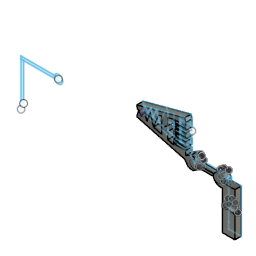
CompliantHands v5 (Autodesk Fusion 360 design; units mm, degrees)
Autodesk Fusion 360 part; units mm, degrees
sketch "Sketch1" plane through (0, 0, 0) normal (0, 1, 0) x (1, 0, 0)
  line L0 (0, 0) -> (19.3185, 5.1764)
  line L1 (0, 0) -> (0.7765, -2.8978)
  line L2 (20.095, 2.2786) -> (19.3185, 5.1764)
  line L3 (0.7765, -2.8978) -> (3.6742, -2.1213)
  line L4 (3.6742, -2.1213) -> (6.572, -1.3449)
  line L5 (6.572, -1.3449) -> (9.4698, -0.5684)
  line L6 (9.4698, -0.5684) -> (12.3676, 0.2081)
  line L7 (12.3676, 0.2081) -> (15.2653, 0.9845)
  line L8 (15.2653, 0.9845) -> (18.1631, 1.761)
  line L9 (20.095, 2.2786) -> (18.1631, 1.761)
  line L10 (12.3676, -8.3553) -> (15.2653, -9.1317)
  line L11 (9.4723, -7.5695) -> (12.3676, -8.3553)
  line L12 (15.2653, -9.1317) -> (18.1631, -9.9082)
  line L13 (0, -8.1472) -> (19.3185, -13.3236)
  line L14 (0.7833, -5.2241) -> (3.6811, -6.0006)
  line L15 (6.5789, -6.777) -> (9.4723, -7.5695)
  line L16 (3.6811, -6.0006) -> (6.5789, -6.777)
  line L17 (20.095, -10.4258) -> (18.1631, -9.9082)
  line L18 (20.095, -10.4258) -> (19.3185, -13.3236)
  line L19 (20.095, 2.2786) -> (20.095, -10.4258)
  line L20 (19.3185, 5.1764) -> (38.637, 10.3528)
  line L21 (20.095, 2.2786) -> (39.4135, 7.455)
  line L22 (39.4135, 7.455) -> (38.637, 10.3528)
  line L23 (20.095, -10.4258) -> (39.4135, -15.6022)
  line L24 (19.3185, -13.3236) -> (38.637, -18.5)
  line L25 (38.637, -18.5) -> (39.4135, -15.6022)
  line L26 (20.095, 2.2786) -> (24.9246, 3.5727)
  line L27 (24.9246, 3.5727) -> (24.9246, -4.0736)
  line L28 (24.9246, -4.0736) -> (24.9246, -11.7199)
  line L29 (20.095, -4.0736) -> (22.095, -4.0736)
  line L30 (24.9246, -4.0736) -> (24.9246, -6.0736)
  line L31 (22.095, -4.0736) -> (24.9246, -6.0736)
  line L32 (24.9246, -4.0736) -> (24.9246, -2.0736)
  line L33 (22.095, -4.0736) -> (24.9246, -2.0736)
  line L34 (39.4135, 7.455) -> (39.4135, 4.8668)
  line L35 (39.4135, 4.8668) -> (29.7542, 4.8668)
  line L36 (39.4135, -15.6022) -> (39.4135, -13.014)
  line L37 (39.4135, -13.014) -> (29.7542, -13.014)
  line L38 (39.4135, 7.455) -> (43.713, 4.9027)
  line L39 (38.637, 10.3528) -> (41.5877, 14.3893)
  line L40 (41.5877, 14.3893) -> (43.713, 4.9027)
  line L41 (39.4135, 0.8668) -> (38.4135, 0.8668)
  line L42 (39.4135, 0.8668) -> (39.4135, 1.8668)
  line L43 (39.4135, 1.8668) -> (29.7542, 1.8668)
  line L44 (29.7542, 1.8668) -> (29.7542, 0.8668)
  line L45 (29.7542, 0.8668) -> (38.4135, 0.8668)
  line L46 (29.7542, 1.8668) -> (29.7542, 4.8668)
  line L47 (29.7542, 4.8668) -> (30.7542, 4.8668)
  line L48 (30.7542, 4.8668) -> (30.7542, 1.8668)
  line L49 (30.7542, 4.8668) -> (39.4135, 4.8668)
  line L50 (39.4135, 4.8668) -> (39.4135, 5.0729)
  circle A0 centre (45.9703, 10.3897) radius 3.4023
  line L51 (46.28, 5.4777) -> (43.713, 4.9027)
  line L52 (41.5877, 14.3893) -> (44.1548, 14.9643)
  spline S0 degree 5 poles (47.6847, 13.3285) (47.6048, 13.4012) (47.4459, 13.5431) (47.2099, 13.746) (46.8999, 13.9959) (46.5209, 14.2717) (46.1512, 14.5071) (45.7919, 14.6983) (45.4434, 14.8421) (45.106, 14.9387) (44.7788, 14.9908) (44.5247, 14.9995) (44.3382, 14.9886) (44.2156, 14.9737) (44.1548, 14.9643) knots 0 0 0 0 0 0 0.1 0.2 0.3 0.4 0.5 0.6 0.7 0.8 0.9 1 1 1 1 1 1
  spline S1 degree 5 poles (48.7311, 8.4013) (48.6822, 8.304) (48.5842, 8.1125) (48.4374, 7.835) (48.2415, 7.4848) (47.9966, 7.0826) (47.7516, 6.7194) (47.5065, 6.3991) (47.2614, 6.1252) (47.0161, 5.8979) (46.7708, 5.7146) (46.5745, 5.6007) (46.4273, 5.5326) (46.3291, 5.4948) (46.28, 5.4777) knots 0 0 0 0 0 0 0.1 0.2 0.3 0.4 0.5 0.6 0.7 0.8 0.9 1 1 1 1 1 1
  circle A1 centre (45.9703, 10.3897) radius 3.3
  line L53 (45.9703, 10.3897) -> (45.9703, 9.3897)
  line L54 (45.9703, 9.3897) -> (70.9703, 9.3897)
  line L55 (70.9703, 9.3897) -> (70.9703, 10.3897)
  line L56 (45.9703, 10.3897) -> (45.9703, 11.3897)
  line L57 (45.9703, 11.3897) -> (70.9703, 11.3897)
  line L58 (70.9703, 11.3897) -> (70.9703, 10.3897)
  line L59 (39.4135, 4.8668) -> (39.4135, 3.8668)
  line L60 (39.4135, 3.8668) -> (30.7542, 3.8668)
  line L61 (39.4135, 1.8668) -> (39.4135, -1.1332)
  line L62 (39.4135, -1.1332) -> (39.4135, -2.1332)
  line L63 (39.4135, -2.1332) -> (29.7542, -2.1332)
  line L64 (29.7542, -2.1332) -> (29.7542, -1.1332)
  line L65 (29.7542, -1.1332) -> (39.4135, -1.1332)
  line L66 (39.4135, -2.1332) -> (38.4135, -2.1332)
  line L67 (38.4135, -2.1332) -> (38.4135, 0.8668)
  line L68 (29.7542, -2.1332) -> (29.7542, -5.1332)
  line L69 (29.7542, -5.1332) -> (39.4135, -5.1332)
  line L70 (39.4135, -5.1332) -> (39.4135, -4.1332)
  line L71 (39.4135, -4.1332) -> (29.7542, -4.1332)
  line L72 (29.7542, -2.1332) -> (30.7542, -2.1332)
  line L73 (30.7542, -2.1332) -> (30.7542, -5.1332)
  line L74 (39.4135, -5.1332) -> (39.4135, -8.1332)
  line L75 (39.4135, -8.1332) -> (29.7542, -8.1332)
  line L76 (29.7542, -8.1332) -> (29.7542, -7.1332)
  line L77 (29.7542, -7.1332) -> (39.4135, -7.1332)
  line L78 (39.4135, -5.1332) -> (38.4135, -5.1332)
  line L79 (38.4135, -5.1332) -> (38.4135, -7.1332)
  line L80 (29.7542, -8.1332) -> (29.7542, -11.1332)
  line L81 (29.7542, -11.1332) -> (39.4135, -11.1332)
  line L82 (39.4135, -11.1332) -> (39.4135, -10.1332)
  line L83 (39.4135, -10.1332) -> (29.7542, -10.1332)
  line L84 (29.7542, -8.1332) -> (30.7542, -8.1332)
  line L85 (30.7542, -8.1332) -> (30.7542, -10.1332)
  line L86 (39.4135, -11.1332) -> (39.4135, -13.014)
  line L87 (39.4135, -11.1332) -> (38.4135, -11.1332)
  line L88 (38.4135, -11.1332) -> (38.4135, -13.014)
  line L89 (68.9703, 41.3897) -> (68.9703, 11.3897)
  line L90 (-98.0297, 41.3897) -> (-98.0297, 46.3897)
  line L91 (-98.0297, 41.3897) -> (-98.0297, 11.3897)
  line L92 (-98.0297, 11.3897) -> (-96.0297, 11.3897)
  line L93 (-96.0297, 11.3897) -> (-96.0297, 41.3897)
  line L94 (-98.0297, 11.3897) -> (-98.0297, 9.3897)
  line L95 (-98.0297, 9.3897) -> (-68.0297, 9.3897)
  line L96 (-68.0297, 9.3897) -> (-68.0297, 11.3897)
  line L97 (-68.0297, 11.3897) -> (-96.0297, 11.3897)
  circle A2 centre (-68.0297, 10.3897) radius 3.3
  line L98 (0.7833, -5.2241) -> (0.9425, -5.2668)
  line L99 (0.7833, -5.2241) -> (0, -8.1472)
  line L100 (1.6898, -5.2715) -> (0.7765, -2.8978)
  line L101 (1.6898, -5.2715) -> (3.6742, -2.1213)
  line L102 (3.769, -2.3626) -> (6.2428, -6.687)
  line L103 (3.769, -2.3626) -> (1.7888, -5.4936)
  line L104 (6.3223, -6.3567) -> (3.8459, -2.0753)
  line L105 (8.0209, -0.9566) -> (6.3223, -6.3567)
  line L106 (8.1279, -1.3139) -> (10.9199, -7.9624)
  line L107 (8.1279, -1.3139) -> (6.4337, -6.7381)
  line L108 (10.9903, -7.6343) -> (13.4864, 0.5078)
  line L109 (10.9903, -7.6343) -> (8.2001, -0.9086)
  line L110 (13.5902, 0.1178) -> (11.0545, -7.9989)
  line L111 (13.5902, 0.1178) -> (17.6214, -9.763)
  line L112 (68.9703, 10.3897) -> (68.9703, 15.3897)
  line L113 (68.9703, 10.3897) -> (68.9703, 5.3897)
  line L114 (68.9703, 10.3897) -> (64.9703, 10.3897)
  circle A3 centre (64.9703, 10.3897) radius 3.4
  circle A4 centre (64.9703, 10.3897) radius 3.3
  spline S2 degree 5 poles (68.9703, 5.3897) (68.8004, 5.3839) (68.4641, 5.3773) (67.9703, 5.3823) (67.3336, 5.4196) (66.5762, 5.5207) (65.8611, 5.6813) (65.192, 5.9068) (64.5715, 6.2007) (63.9983, 6.5614) (63.4693, 6.9844) (63.0786, 7.3687) (62.8027, 7.6811) (62.6263, 7.8999) (62.54, 8.012) knots 0 0 0 0 0 0 0.1 0.2 0.3 0.4 0.5 0.6 0.7 0.8 0.9 1 1 1 1 1 1
  spline S3 degree 5 poles (68.9703, 15.3897) (68.7911, 15.4037) (68.4369, 15.4261) (67.9187, 15.4426) (67.2541, 15.4299) (66.4705, 15.3522) (65.7385, 15.2068) (65.0627, 14.9875) (64.4466, 14.6899) (63.8891, 14.3155) (63.3861, 13.8693) (63.0241, 13.4595) (62.7739, 13.1241) (62.6164, 12.8884) (62.54, 12.7674) knots 0 0 0 0 0 0 0.1 0.2 0.3 0.4 0.5 0.6 0.7 0.8 0.9 1 1 1 1 1 1
  line L115 (68.9703, 5.3897) -> (70.9703, 9.3897)
  line L116 (68.9703, 11.3897) -> (73.9703, 11.3897)
  line L117 (68.9703, 41.3897) -> (68.9703, 46.3897)
  line L118 (68.9703, 46.3897) -> (78.9703, 46.3897)
  line L119 (78.9703, 46.3897) -> (78.9703, 11.3897)
  line L120 (78.9703, 11.3897) -> (73.9703, 11.3897)
  line L121 (73.9703, 28.6756, 0) -> (73.9703, 28.6756, -2.5)
  spline S4 degree 5 poles (78.9703, 28.5551, -2.5) (78.7318, 28.5315, -2.5) (78.279, 28.4726, -2.5) (77.672, 28.3491, -2.5) (77.0087, 28.1138, -2.5) (76.4256, 27.7009, -2.5) (76.087, 27.1721, -2.5) (75.9801, 26.5373, -2.5) (76.0744, 25.8179, -2.5) (76.3133, 25.051, -2.5) (76.6223, 24.2824, -2.5) (76.9143, 23.5589, -2.5) (77.099, 22.9217, -2.5) (77.0823, 22.3974, -2.5) (76.7907, 21.9946, -2.5) (76.1933, 21.7173, -2.5) (75.4616, 21.595, -2.5) (74.7708, 21.5585, -2.5) (74.2476, 21.5584, -2.5) (73.9703, 21.5645, -2.5) knots 0 0 0 0 0 0 0.06666667 0.13333333 0.2 0.26666667 0.33333333 0.4 0.46666667 0.53333333 0.6 0.66666667 0.73333333 0.8 0.86666667 0.93333333 1 1 1 1 1 1
  line L122 (76.9946, 23.5633, -2.5) -> (77.1193, 22.1919, -2.5)
  spline S5 degree 5 poles (68.9703, 28.6756, -2.5) (69.2439, 28.6361, -2.5) (69.7595, 28.5449, -2.5) (70.4386, 28.3716, -2.5) (71.1554, 28.0672, -2.5) (71.7402, 27.5669, -2.5) (72.0279, 26.9539, -2.5) (72.0496, 26.2446, -2.5) (71.859, 25.4662, -2.5) (71.5414, 24.6622, -2.5) (71.2024, 23.8856, -2.5) (70.9504, 23.1892, -2.5) (70.8801, 22.6165, -2.5) (71.057, 22.1933, -2.5) (71.4979, 21.916, -2.5) (72.1744, 21.7582, -2.5) (73.0259, 21.6851, -2.5) (73.9703, 21.6656, -2.5) (74.9148, 21.6851, -2.5) (75.7663, 21.7582, -2.5) (76.4428, 21.916, -2.5) (76.8837, 22.1933, -2.5) (77.0606, 22.6165, -2.5) (76.9903, 23.1892, -2.5) (76.7383, 23.8856, -2.5) (76.3993, 24.6622, -2.5) (76.0817, 25.4662, -2.5) (75.8911, 26.2446, -2.5) (75.9128, 26.9539, -2.5) (76.2005, 27.5669, -2.5) (76.7853, 28.0672, -2.5) (77.5021, 28.3716, -2.5) (78.1812, 28.5449, -2.5) (78.6968, 28.6361, -2.5) (78.9703, 28.6756, -2.5) knots 0 0 0 0 0 0 0.03333333 0.06666667 0.1 0.13333333 0.16666667 0.2 0.23333333 0.26666667 0.3 0.33333333 0.36666667 0.4 0.43333333 0.46666667 0.5 0.53333333 0.56666667 0.6 0.63333333 0.66666667 0.7 0.73333333 0.76666667 0.8 0.83333333 0.86666667 0.9 0.93333333 0.96666667 1 1 1 1 1 1
  line L123 (73.9703, 22.5079, -2.5) -> (76.9703, 22.5079, -2.5)
  line L124 (73.9703, 28.6756, -2.5) -> (73.9703, 21.6756, -2.5)
  line L125 (73.9703, 22.5079, -2.5) -> (70.9703, 22.5079, -2.5)
  line L126 (73.9703, 26.0373, -2.5) -> (71.9703, 26.0373, -2.5)
  line L127 (73.9703, 26.0373, -2.5) -> (75.9703, 26.0373, -2.5)
  line L128 (68.9703, 28.6756, -2.5) -> (78.9703, 28.6756, -2.5)
  spline S6 degree 5 poles (68.9703, 28.5551, -2.5) (69.2228, 28.5188, -2.5) (69.7009, 28.4362, -2.5) (70.338, 28.2817, -2.5) (71.0261, 28.0143, -2.5) (71.6143, 27.577, -2.5) (71.9338, 27.039, -2.5) (72.0011, 26.4092, -2.5) (71.8545, 25.7061, -2.5) (71.5633, 24.9626, -2.5) (71.217, 24.2196, -2.5) (70.9128, 23.52, -2.5) (70.7448, 22.9025, -2.5) (70.7926, 22.3956, -2.5) (71.1079, 22.0101, -2.5) (71.7206, 21.7442, -2.5) (72.4611, 21.6211, -2.5) (73.1599, 21.5753, -2.5) (73.6896, 21.5647, -2.5) (73.9703, 21.5645, -2.5) knots 0 0 0 0 0 0 0.06666667 0.13333333 0.2 0.26666667 0.33333333 0.4 0.46666667 0.53333333 0.6 0.66666667 0.73333333 0.8 0.86666667 0.93333333 1 1 1 1 1 1
  line L129 (72.0248, 21.5663, -2.5) -> (75.9159, 21.5627, -2.5)
  line L130 (78.9703, 28.6756, -2.5) -> (78.9703, 28.5551, -2.5)
  line L131 (68.9703, 28.6756, -2.5) -> (68.9703, 28.5551, -2.5)
  line L132 (73.9703, 21.6756, -2.5) -> (73.9703, 21.5645, -2.5)
  line L133 (68.9703, 28.5551, -2.5) -> (78.9703, 28.5551, -2.5)
  point P0 (45.6581, 14.7479)
  point P1 (47.3897, 6.2744)
  point P2 (65.0929, 5.97)
  point P3 (64.933, 14.9075)
  point P4 (70.7943, 22.8776)
  point P5 (71.9454, 26.3514)
  point P6 (77.0569, 22.8776)
  point P7 (76.0301, 26.5116)
  dimension "d1" = 20
  dimension "d2" = 3
  dimension "d3" = 3
  dimension "d4" = 3
  dimension "d5" = 3
  dimension "d6" = 3
  dimension "d7" = 3
  dimension "d8" = 3
  dimension "d15" = 20
  dimension "d17" = 3
  dimension "d18" = 3
  dimension "d19" = 3
  dimension "d20" = 3
  dimension "d21" = 3
  dimension "d22" = 3
  dimension "d23" = 20
  dimension "d24" = 20
  dimension "d26" = 20
  dimension "d27" = 5
  dimension "d28" = 2
  dimension "d29" = 2
  dimension "d30" = 2
  dimension "d51" = 5
  dimension "d52" = 5
  dimension "d59" = 1
  dimension "d60" = 3
  dimension "d61" = 1
  dimension "d67" = 6.6
  dimension "d68" = 25
  dimension "d69" = 1
  dimension "d70" = 1
  dimension "d83" = 1
  dimension "d84" = 3
  dimension "d85" = 1
  dimension "d86" = 1
  dimension "d87" = 1
  dimension "d88" = 3
  dimension "d89" = 1
  dimension "d90" = 1
  dimension "d91" = 3
  dimension "d92" = 1
  dimension "d93" = 1
  dimension "d94" = 3
  dimension "d95" = 1
  dimension "d96" = 1
  dimension "d97" = 1
  dimension "d102" = 2
  dimension "d103" = 2
  dimension "d104" = 30
  dimension "d105" = 2
  dimension "d106" = 6.6
  dimension "d112" = 5
  dimension "d113" = 5
  dimension "d114" = 4
  dimension "d115" = 6.8
  dimension "d116" = 6.6
  dimension "d117" = 5
  dimension "d122" = 10
  dimension "d130" = 2.5
  dimension "d131" = 7
  dimension "d132" = 3
  dimension "d133" = 3
  dimension "d134" = 2
  dimension "d135" = 2
  constraint coincident L0.start L1.start
  constraint perpendicular L0 L1
  constraint perpendicular L0 L2
  constraint perpendicular L1 L3
  constraint perpendicular L1 L4
  constraint perpendicular L2 L9
  constraint perpendicular L13 L18
  constraint perpendicular L17 L18
  constraint vertical L19
  constraint perpendicular L2 L20
  constraint perpendicular L2 L21
  constraint perpendicular L18 L23
  constraint perpendicular L18 L24
  constraint perpendicular L23 L25
  constraint perpendicular L2 L26
  constraint parallel L19 L27
  constraint coincident L23 L28.end
  constraint parallel L27 L28
  constraint midpoint L19 L29.start
  constraint perpendicular L19 L29
  constraint parallel L28 L30
  constraint coincident L27 L32.end
  constraint parallel L32 L34
  constraint midpoint L21 L35.end
  constraint perpendicular L34 L35
  constraint perpendicular L35 L36
  constraint midpoint L23 L37.end
  constraint perpendicular L36 L37
  constraint perpendicular L41 L42
  constraint perpendicular L43 L44
  constraint perpendicular L43 L46
  constraint perpendicular L44 L47
  constraint coincident L43 L48.end
  constraint perpendicular L43 L48
  constraint perpendicular L34 L49
  constraint coincident L34 L50.end
  constraint perpendicular L35 L50
  constraint coincident A0 S1.start
  constraint coincident A0 S0.start
  constraint perpendicular L40 L51
  constraint concentric A0 A1
  constraint coincident A0.centre A1.centre
  constraint perpendicular L53 L54
  constraint perpendicular L55 L57
  constraint perpendicular L35 L59
  constraint coincident L48 L60.end
  constraint perpendicular L48 L60
  constraint perpendicular L43 L61
  constraint perpendicular L43 L62
  constraint perpendicular L44 L63
  constraint perpendicular L45 L64
  constraint perpendicular L62 L65
  constraint coincident L63 L66.end
  constraint perpendicular L45 L67
  constraint perpendicular L63 L68
  constraint perpendicular L62 L69
  constraint perpendicular L66 L70
  constraint coincident L68 L71.end
  constraint perpendicular L68 L71
  constraint perpendicular L68 L72
  constraint coincident L69 L73.end
  constraint perpendicular L69 L73
  constraint perpendicular L69 L74
  constraint perpendicular L70 L75
  constraint perpendicular L75 L76
  constraint perpendicular L70 L77
  constraint perpendicular L74 L78
  constraint coincident L77 L79.end
  constraint perpendicular L77 L79
  constraint perpendicular L75 L80
  constraint perpendicular L80 L81
  constraint perpendicular L75 L82
  constraint coincident L80 L83.end
  constraint perpendicular L80 L83
  constraint perpendicular L76 L84
  constraint coincident L83 L85.end
  constraint perpendicular L83 L85
  constraint perpendicular L37 L86
  constraint perpendicular L86 L87
  constraint coincident L37 L88.end
  constraint perpendicular L37 L88
  constraint coincident L57 L89.end
  constraint perpendicular L57 L89
  constraint vertical L90
  constraint perpendicular L91 L92
  constraint perpendicular L92 L94
  constraint perpendicular L94 L95
  constraint perpendicular L95 L96
  constraint coincident L14 L98.end
  constraint coincident L14 L103.end
  constraint coincident L16 L102.end
  constraint midpoint L5 L105.start
  constraint coincident L16 L107.end
  constraint midpoint L11 L106.end
  constraint coincident L5 L109.end
  constraint coincident L7 L108.end
  constraint coincident L11 L110.end
  constraint coincident L12 L111.end
  constraint coincident L4 L104.end
  constraint coincident L89 L112.end
  constraint perpendicular L54 L113
  constraint perpendicular L112 L114
  constraint coincident L114.end A3.centre
  constraint concentric A3 A4
  constraint coincident A3 S2.end
  constraint coincident A3 S3.end
  constraint perpendicular L58 L116
  constraint parallel L89 L117
  constraint perpendicular L117 L118
  constraint perpendicular L116 L119
  measures "d1" distance of L0.start L0.end
  measures "d2" distance of L0.start L1.end
  measures "d3" distance of L1.end L3.end
  measures "d4" distance of L3.end L4.end
  measures "d5" distance of L4.end L5.end
  measures "d6" distance of L5.end L6.end
  measures "d7" distance of L6.end L7.end
  measures "d8" distance of L7.end L8.end
  measures "d15" distance of L13.start L13.end
  measures "d17" distance of L14.start L14.end
  measures "d18" distance of L14.end L15.start
  measures "d19" distance of L11.start L15.start
  measures "d20" distance of L10.start L11.start
  measures "d21" distance of L10.end L10.start
  measures "d22" distance of L10.end L12.end
  measures "d23" distance of L0.end L20.end
  measures "d24" distance of L2.start L21.end
  measures "d26" distance of L13.end L24.end
  measures "d27" distance of L2.start L26.end
  measures "d28" distance of L29.start L29.end
  measures "d29" distance of L27.end L30.end
  measures "d30" distance of L27.end L32.end
  measures "d51" distance of L21.end L38.end
  measures "d52" distance of L20.end L39.end
  measures "d59" distance of L41.start L42.end
  measures "d60" distance of L43.end L35.end
  measures "d61" distance of L35.end L47.end
  measures "d67" diameter of A1
  measures "d68" distance of A0.centre L55.end
  measures "d69" distance of A0.centre L53.end
  measures "d70" distance of A0.centre L56.end
  measures "d83" distance of L34.end L59.end
  measures "d84" distance of L42.end L61.end
  measures "d85" distance of L61.end L62.end
  measures "d86" distance of L63.end L64.end
  measures "d87" distance of L62.end L66.end
  measures "d88" distance of L63.end L68.end
  measures "d89" distance of L69.end L70.end
  measures "d90" distance of L63.end L72.end
  measures "d91" distance of L69.end L74.end
  measures "d92" distance of L75.end L76.end
  measures "d93" distance of L69.end L78.end
  measures "d94" distance of L75.end L80.end
  measures "d95" distance of L81.end L82.end
  measures "d96" distance of L75.end L84.end
  measures "d97" distance of L81.end L87.end
  measures "d102" distance of L91.end L92.end
  measures "d103" distance of L91.end L94.end
  measures "d104" distance of L94.end L95.end
  measures "d105" distance of L95.end L96.end
  measures "d106" diameter of A2
  measures "d112" distance of L112.start L112.end
  measures "d113" distance of L112.start L113.end
  measures "d114" distance of L112.start L114.end
  measures "d115" diameter of A3
  measures "d116" diameter of A4
  measures "d117" distance of L89.end L116.end
  measures "d122" distance of L117.end L118.end
extrude "Extrude1" add sketch "Sketch1" against normal blind 5 contours L0 L1 L2 L3 L4 L5 L6 L7 L8 L9 | L2 L20 L21 L22 L26 | L3 L100 L101 | L19 L21 L26 L27 L29 L33 | L19 L23 L28 L29 L31 | L21 L34 L35 L47 L49 L50 | L4 L5 L104 L105 | L10 L11 L12 L13 L14 L15 L16 L17 L18 L98 L99 | L18 L23 L24 L25 | L35 L43 L46 L47 L48 | L5 L6 L7 L108 L109 | L35 L48 L49 L59 L60 | L41 L42 L43 L44 L45 L61 | L10 L11 L12 L110 L111 | L23 L36 L37 | L37 L81 L86 L87 L88 | L41 L61 L65 L67 | L80 L81 L82 L83 L87 | L63 L64 L65 L67 L72 | L62 L63 L65 L66 L67 | L11 L15 L16 L106 L107 | L14 L16 L102 L103 | L75 L80 L83 L84 L85 | L63 L68 L71 L72 L73 | L74 L75 L76 L77 L84 | L68 L69 L71 L73 | L69 L70 L71 L73 L78 | L69 L74 L77 L78 L79 makes body 1
extrude "Extrude2" add sketch "Sketch1" against normal blind 5 contours L22 L38 L39 L40 | L40 A0 L52 S0 | L40 A0 L51 S1 | L57 L89 L112 A3 S3 | L54 L113 A3 S2 | L57 L112 L114 A3 | L54 L113 L114 A3 | L54 L113 L115 bodies 1 makes body 2 at (66.8464, -1.6667, -7.5541)
extrude "Extrude3" add sketch "Sketch1" against normal blind 0.5 contours A0 A1 L54 L57 | A0 A1 L54 L57 | A1 L53 L54 L56 L57 | A1 L53 L54 L56 L57 | L57 A3 A4 | L54 L57 A3 A4 | L54 A3 A4 | L57 A4 | L54 L57 A4 | L54 A4 | L57 L114 A3 A4 | L54 L114 A3 A4 bodies 1 2
extrude "Extrude4" add sketch "Sketch1" along normal blind -5 and the other way blind 4.5 contours A0 A1 L54 L57 | A0 A1 L54 L57 | A1 L53 L54 L56 L57 | A1 L53 L54 L56 L57 | L57 A3 A4 | L54 L57 A3 A4 | L54 A3 A4 | L57 A4 | L54 L57 A4 | L54 A4 | L57 L114 A3 A4 | L54 L114 A3 A4 bodies 1 2
extrude "Extrude5" add sketch "Sketch1" along normal blind -4.4 and the other way blind 0.6 contours A0 L54 L57 A3 | A0 A1 L54 L57 | A1 L53 L54 L56 L57 | A1 L53 L54 L56 L57 | L54 L57 A3 A4 | L57 A4 | L54 L57 A4 | L54 A4 | L57 L112 L114 A3 | L54 L113 L114 A3 | L54 L55 L57 L58 L112 L113 L116 picked at (49.1795, 11.2806) bodies 2 makes body 3 at (63.7952, -0.6, -9.9702)
extrude "Extrude6" add sketch "Sketch1" against normal blind 5 contours L57 L89 L112 L116 L117 L118 L119 L120 | L54 L55 L57 L58 L112 L113 L116 bodies 2
revolve "Revolve1" cut sketch "Sketch1" angle 360 about axis through (73.9703, -2.5, -28.6756) along (0, 0, 1) contours S5 L130 L133 | S4 S5 L129 L132 L133 | S5 L124 L128 L133 | S5 L124 L127 L133 | S4 L129 | S5 L123 L124 L127 | S5 L123 L124 in plane through (0, -2.5, 0) normal (0, 1, 0) picked at (77.0788, -2.5, -28.6354) bodies 2
extrude "Extrude7" cut sketch "Sketch1" along normal mid plane 9 contours S5 L130 L133 | S5 L124 L128 L133 | S5 L124 L128 L133 | S5 L131 L133 in plane through (0, -2.5, 0) normal (0, 1, 0) bodies 2 makes body 4 at (72.3037, 0, -40.485)
revolve "Revolve2" add sketch "Sketch1" angle 360 about axis through (73.9703, -2.5, -28.6756) along (0, 0, 1) contours S5 L124 L128 L133 | S5 L124 L127 L133 | S5 L123 L124 L127 | S5 L123 L124 in plane through (0, -2.5, 0) normal (0, 1, 0) picked at (77.0788, -2.5, -28.6354) bodies 4
extrude "Extrude8" cut sketch "Sketch1" along normal blind 3 contours L57 L89 L112 L116 L117 L118 L119 L120 bodies 4
extrude "Extrude9" cut sketch "Sketch1" along normal blind -8 and the other way blind 5 contours L57 L89 L112 L116 L117 L118 L119 L120 bodies 4
named bodies: "Clamp", "JointJoiner", "Joint", "RotJoint"
